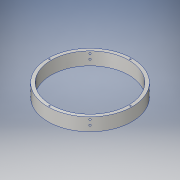
# Autodesk Inventor part: ontelMounting
Saved by Autodesk Inventor 2016 (Build 200138000, 138)
## iProperties
Created: 2015-12-10
Part Number: ontelMounting
Material: Aluminum 6061
Document SubType Name: Modeling
Designer: Dave
Density: 2.7 g/cm^3
Appearance: Aluminum - Flat
Mass: 1717.63 g
Surface Area: 1312.48 cm^2
Volume: 636.161 cm^3
Author: Dave
Autodesk Inventor part; units mm, degrees
ref_plane "YZ Plane" through (0, 0, 0) normal (1, 0, 0) x (0, 1, 0)
ref_plane "XZ Plane" through (0, 0, 0) normal (0, 1, 0) x (-1, 0, 0)
ref_plane "XY Plane" through (0, 0, 0) normal (0, 0, 1) x (1, 0, 0)
sketch "Sketch1" plane through (0, 0, 0) normal (0, 1, 0) x (-1, 0, 0)
  circle A0 centre (0, 0) radius 165.1
  circle A1 centre (0, 0) radius 152.4
  dimension "d0" = 330.2
  dimension "d1" = 12.7
  constraints: 2 centre point, 1 coincident
  measures "d0" diameter of A0
  measures "d1" radial gap between concentric circles of A1 A0
extrude "Extrusion1" add sketch "Sketch1" along normal blind 50.8
sketch "Sketch2" plane through (0, 50.8, 0) normal (0, 1, 0) x (1, 0, 0)
  circle A0 centre (0, -158.75) radius 3.8282
  point P0 (0, 0)
  dimension "d4" = 158.75
  constraints: 1 centre point
  measures "d4" distance of A0.centre point (0, 0)
hole "Hole1" at (0, 50.8, 158.75) direction (0, -1, 0) diameter 4.9784 end through all thread size "1/4-20 UNC" class "2B" standard "ANSI Unified Screw Threads"
pattern_circular "Circular Pattern1" count 4 over 360 about axis through (0, -10, 0) along (0, 1, 0) of "Hole1"
sketch "Sketch3" plane through (0, 50.8, 0) normal (0, 1, 0) x (1, 0, 0)
  line L0 (0, 0) -> (-167.6109, 167.6109) construction
  line L1 (0, 0) -> (237.0376, 0) construction
  circle A0 centre (0, 0) radius 165.1 projected
  point P0 (-116.7433, 116.7433)
  dimension "d15" = 135
  constraints: 4 end point, 1 equal length, 1 horizontal, 1 point on line, 2 other
  measures "d15" angle of L1 L0
ref_plane "Work Plane1" through (-116.7433, 50.8, -116.7433) normal (-0.7071068, 0, -0.7071068) x (0, -1, 0)
sketch "Sketch4" plane through (-116.7433, 50.8, -116.7433) normal (-0.7071068, 0, -0.7071068) x (0, -1, 0)
  circle A0 centre (9.525, 0) radius 2.9411
  circle A1 centre (28.575, 0) radius 3.3282
  line L0 (0, 165.1) -> (0, -165.1) projected
  point P0 (50.8, 0)
  dimension "d16" = 9.525
  dimension "d17" = 19.05
  constraints: 2 centre point
  measures "d16" distance from line of A0.centre L0
  measures "d17" distance of A1.centre A0.centre
hole "Hole2" at (-116.7433, 22.225, -116.7433) at (-116.7433, 41.275, -116.7433) direction (0.7071068, 0, 0.7071068) diameter 6.5278 end through all clearance for "Flat Head Machine Screw (82)" size "1/4" standard "Ansi Unified Screw Threads"
pattern_circular "Circular Pattern2" count 4 over 360 about axis through (0, -10, 0) along (0, 1, 0) of "Hole2"
body "Solid1"
